saddle_coupon (Autodesk Fusion 360 design; units mm, degrees)
part number: 2026-09-02-15-56-22-744
Autodesk Fusion 360 part; units mm, degrees
sketch "Coupon chord" plane through (0, 0, 0) normal (0, 1, 0) x (1, 0, 0)
  line L0 (70, -76) -> (150, -76)
  line L1 (150, -76) -> (150, -90)
  line L2 (150, -90) -> (70, -90)
  line L3 (70, -90) -> (70, -76)
extrude "Coupon chord (1)" add sketch "Coupon chord" along normal mid plane 8
sketch "Saddle boss x=70" plane through (0, 0, 0) normal (0, 1, 0) x (1, 0, 0)
  circle A0 centre (70, -90) radius 22.7
extrude "Saddle boss x=70 (1)" add sketch "Saddle boss x=70" along normal mid plane 8
sketch "Saddle boss x=150" plane through (0, 0, 0) normal (0, 1, 0) x (1, 0, 0)
  circle A0 centre (150, -90) radius 22.7
extrude "Saddle boss x=150 (1)" add sketch "Saddle boss x=150" along normal mid plane 8
sketch "Rod pocket x=70" plane through (0, 0, 0) normal (0, 1, 0) x (1, 0, 0)
  circle A0 centre (70, -90) radius 17.1
extrude "Rod pocket x=70 (1)" cut sketch "Rod pocket x=70" along normal mid plane 18
sketch "Drop-in opening x=70" plane through (0, 0, 0) normal (0, 1, 0) x (1, 0, 0)
  line L0 (52.9, -90) -> (87.1, -90)
  line L1 (87.1, -90) -> (87.1, -117.7)
  line L2 (87.1, -117.7) -> (52.9, -117.7)
  line L3 (52.9, -117.7) -> (52.9, -90)
extrude "Drop-in opening x=70 (1)" cut sketch "Drop-in opening x=70" along normal mid plane 18
sketch "Rod pocket x=150" plane through (0, 0, 0) normal (0, 1, 0) x (1, 0, 0)
  circle A0 centre (150, -90) radius 17.1
extrude "Rod pocket x=150 (1)" cut sketch "Rod pocket x=150" along normal mid plane 18
sketch "Drop-in opening x=150" plane through (0, 0, 0) normal (0, 1, 0) x (1, 0, 0)
  line L0 (132.9, -90) -> (167.1, -90)
  line L1 (167.1, -90) -> (167.1, -117.7)
  line L2 (167.1, -117.7) -> (132.9, -117.7)
  line L3 (132.9, -117.7) -> (132.9, -90)
extrude "Drop-in opening x=150 (1)" cut sketch "Drop-in opening x=150" along normal mid plane 18
equation "bracketWidth = 24.0 mm" comment "drives the model; safe to edit live in Fusion"
equation "couponWidth = 8.0 mm" comment "drives the model; safe to edit live in Fusion"
equation "hookTabWidth = 2.4 mm" comment "drives the model; safe to edit live in Fusion"
equation "slotHeight = 19.05 mm" comment "reference only â edit scripts/build_rod_bracket.py and rebuild"
equation "slotPitchVertical = 25.4 mm" comment "drives the model; safe to edit live in Fusion"
equation "slotWidth = 3.2 mm" comment "reference only â edit scripts/build_rod_bracket.py and rebuild"
equation "faceMetalThickness = 2.0 mm" comment "drives the model; safe to edit live in Fusion"
equation "hookThroat = faceMetalThickness + 1.8 mm" comment "drives the model; safe to edit live in Fusion"
equation "hookNeckHeight = 5.0 mm" comment "drives the model; safe to edit live in Fusion"
equation "hookLipThickness = 4.5 mm" comment "drives the model; safe to edit live in Fusion"
equation "hookLipDrop = 12.0 mm" comment "drives the model; safe to edit live in Fusion"
equation "plateThickness = 6.0 mm" comment "reference only â edit scripts/build_rod_bracket.py and rebuild"
equation "plateHeight = 90.0 mm" comment "reference only â edit scripts/build_rod_bracket.py and rebuild"
equation "gaugePlateThickness = 5.0 mm" comment "reference only â edit scripts/build_rod_bracket.py and rebuild"
equation "rodOuterDiameter = 33.4 mm" comment "reference only â edit scripts/build_rod_bracket.py and rebuild"
equation "saddleClearance = 0.8 mm" comment "reference only â edit scripts/build_rod_bracket.py and rebuild"
equation "saddleWall = 6.0 mm" comment "reference only â edit scripts/build_rod_bracket.py and rebuild"
equation "rearRodStandoff = 70.0 mm" comment "reference only â edit scripts/build_rod_bracket.py and rebuild"
equation "rodSpacing = 80.0 mm" comment "reference only â edit scripts/build_rod_bracket.py and rebuild"
equation "memberWidth = 14.0 mm" comment "reference only â edit scripts/build_rod_bracket.py and rebuild"
equation "hookLipChamfer = 1.5 mm" comment "drives the model; safe to edit live in Fusion"
equation "topHookNeckTop = 88.0 mm" comment "drives the model; safe to edit live in Fusion"
equation "hookRows = 4" comment "drives the model; safe to edit live in Fusion"
equation "d38 = couponWidth"
equation "d40 = couponWidth"
equation "d42 = couponWidth"
equation "d44 = couponWidth + 10 mm"
equation "d46 = couponWidth + 10 mm"
equation "d48 = couponWidth + 10 mm"
equation "d50 = couponWidth + 10 mm"
named bodies: "saddle_coupon"
